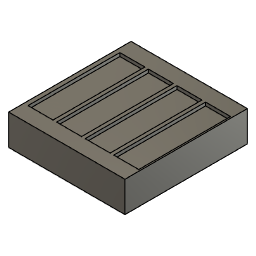
両端 v1 (Autodesk Fusion 360 design; units mm, degrees)
Autodesk Fusion 360 part; units mm, degrees
sketch "スケッチ1" plane through (0, 0, 0) normal (0, 1, 0) x (1, 0, 0)
  line L0 (0, 0) -> (-114, 0)
  line L1 (-114, 0) -> (-114, 120)
  line L2 (-114, 120) -> (0, 120)
  line L3 (0, 120) -> (0, 0)
  dimension "d1" = 114
  dimension "d2" = 120
  constraint horizontal L0
  constraint vertical L1
  constraint horizontal L2
  constraint vertical L3
  constraint coincident L0.start L3.end
  measures "d1" distance of L0.start L0.end
  measures "d2" distance of L0.start L2.end
extrude "押し出し1" add sketch "スケッチ1" along normal blind 40
sketch "スケッチ2" plane through (0, 40, 0) normal (0, 1, 0) x (-1, 0, 0)
  line L0 (0, -120) -> (114, -120)
  line L1 (114, -120) -> (114, 0)
  line L2 (114, 0) -> (0, 0)
  line L3 (0, 0) -> (0, -120)
  line L4 (0, -105) -> (1.5, -105)
  line L5 (1.5, -105) -> (1.5, -15)
  line L6 (1.5, -15) -> (0, -15)
  line L7 (0, -15) -> (0, -105)
  line L8 (1.5, -105) -> (26, -105)
  line L9 (26, -105) -> (26, -15)
  line L10 (26, -15) -> (1.5, -15)
  line L11 (1.5, -15) -> (1.5, -105)
  line L12 (26, -105) -> (29.5, -105)
  line L13 (29.5, -105) -> (29.5, -15)
  line L14 (29.5, -15) -> (26, -15)
  line L15 (26, -15) -> (26, -105)
  line L16 (29.5, -105) -> (54, -105)
  line L17 (54, -105) -> (54, -15)
  line L18 (54, -15) -> (29.5, -15)
  line L19 (29.5, -15) -> (29.5, -105)
  line L20 (54, -105) -> (57.5, -105)
  line L21 (57.5, -105) -> (57.5, -15)
  line L22 (57.5, -15) -> (54, -15)
  line L23 (54, -15) -> (54, -105)
  line L24 (57.5, -105) -> (82, -105)
  line L25 (82, -105) -> (82, -15)
  line L26 (82, -15) -> (57.5, -15)
  line L27 (57.5, -15) -> (57.5, -105)
  line L28 (82, -105) -> (85.5, -105)
  line L29 (85.5, -105) -> (85.5, -15)
  line L30 (85.5, -15) -> (82, -15)
  line L31 (82, -15) -> (82, -105)
  line L32 (85.5, -105) -> (110, -105)
  line L33 (110, -105) -> (110, -15)
  line L34 (110, -15) -> (85.5, -15)
  line L35 (85.5, -15) -> (85.5, -105)
  line L36 (110, -105) -> (114, -105)
  line L37 (114, -105) -> (114, -15)
  line L38 (114, -15) -> (110, -15)
  line L39 (110, -15) -> (110, -105)
  dimension "d5" = 1.5
  dimension "d6" = 90
  dimension "d7" = 24.5
  dimension "d8" = 90
  dimension "d9" = 3.5
  dimension "d10" = 90
  dimension "d11" = 24.5
  dimension "d12" = 90
  dimension "d13" = 3.5
  dimension "d14" = 90
  dimension "d15" = 24.5
  dimension "d16" = 90
  dimension "d17" = 3.5
  dimension "d18" = 90
  dimension "d19" = 24.5
  dimension "d20" = 90
  dimension "d21" = 4
  dimension "d22" = 90
  constraint horizontal L4
  constraint vertical L5
  constraint horizontal L6
  constraint vertical L7
  constraint coincident L3 L4.start
  constraint horizontal L8
  constraint vertical L9
  constraint horizontal L10
  constraint vertical L11
  constraint horizontal L12
  constraint vertical L13
  constraint horizontal L14
  constraint vertical L15
  constraint horizontal L16
  constraint vertical L17
  constraint horizontal L18
  constraint vertical L19
  constraint horizontal L20
  constraint vertical L21
  constraint horizontal L22
  constraint vertical L23
  constraint horizontal L24
  constraint vertical L25
  constraint horizontal L26
  constraint vertical L27
  constraint horizontal L28
  constraint vertical L29
  constraint horizontal L30
  constraint vertical L31
  constraint horizontal L32
  constraint vertical L33
  constraint horizontal L34
  constraint vertical L35
  constraint horizontal L36
  constraint vertical L37
  constraint horizontal L38
  constraint vertical L39
  measures "d5" distance of L4.start L4.end
  measures "d6" distance of L4.start L6.end
  measures "d7" distance of L4.end L8.end
  measures "d8" distance of L4.end L5.end
  measures "d9" distance of L8.end L12.end
  measures "d10" distance of L8.end L9.end
  measures "d11" distance of L12.end L16.end
  measures "d12" distance of L12.end L13.end
  measures "d13" distance of L16.end L20.end
  measures "d14" distance of L16.end L17.end
  measures "d15" distance of L20.end L24.end
  measures "d16" distance of L20.end L21.end
  measures "d17" distance of L24.end L28.end
  measures "d18" distance of L24.end L25.end
  measures "d19" distance of L28.end L32.end
  measures "d20" distance of L28.end L29.end
  measures "d21" distance of L32.end L36.end
  measures "d22" distance of L32.end L33.end
extrude "押し出し2" cut sketch "スケッチ2" against normal blind 3 contours L29 L32 L33 L34 L35 L39
sketch "スケッチ3" plane through (0, 40, 0) normal (0, 1, 0) x (-1, 0, 0)
  line L0 (110, -105) -> (85.5, -105)
  line L1 (85.5, -105) -> (85.5, -15)
  line L2 (85.5, -15) -> (110, -15)
  line L3 (110, -15) -> (110, -105)
  line L4 (0, -120) -> (114, -120)
  line L5 (114, -120) -> (114, 0)
  line L6 (114, 0) -> (0, 0)
  line L7 (0, 0) -> (0, -120)
  line L8 (0, -105) -> (1.5, -105)
  line L9 (1.5, -105) -> (1.5, -15)
  line L10 (1.5, -15) -> (0, -15)
  line L11 (0, -15) -> (0, -105)
  line L12 (1.5, -105) -> (26, -105)
  line L13 (26, -105) -> (26, -15)
  line L14 (26, -15) -> (1.5, -15)
  line L15 (1.5, -15) -> (1.5, -105)
  dimension "d25" = 1.5
  dimension "d26" = 90
  dimension "d27" = 24.5
  dimension "d28" = 90
  constraint horizontal L8
  constraint vertical L9
  constraint horizontal L10
  constraint vertical L11
  constraint coincident L7 L8.start
  constraint horizontal L12
  constraint vertical L13
  constraint horizontal L14
  constraint vertical L15
  measures "d25" distance of L8.start L8.end
  measures "d26" distance of L8.start L10.end
  measures "d27" distance of L8.end L12.end
  measures "d28" distance of L8.end L9.end
extrude "押し出し3" cut sketch "スケッチ3" against normal blind 3 contours L9 L12 L13 L14 L15
extrude "押し出し4" cut 1 faces at (-93.6667, 37, -45) along direction (0, -1, 0) blind 0.3
extrude "押し出し5" cut 1 faces at (-9.6667, 37, -45) along direction (0, -1, 0) blind 0.3
sketch "スケッチ4" plane through (0, 40, 0) normal (0, 1, 0) x (-1, 0, 0)
  line L0 (26, -105) -> (1.5, -105)
  line L1 (1.5, -105) -> (1.5, -15)
  line L2 (1.5, -15) -> (26, -15)
  line L3 (26, -15) -> (26, -105)
  line L4 (110, -105) -> (85.5, -105)
  line L5 (85.5, -105) -> (85.5, -15)
  line L6 (85.5, -15) -> (110, -15)
  line L7 (110, -15) -> (110, -105)
  line L8 (0, -120) -> (114, -120)
  line L9 (114, -120) -> (114, 0)
  line L10 (114, 0) -> (0, 0)
  line L11 (0, 0) -> (0, -120)
  line L12 (26, -105) -> (29.5, -105)
  line L13 (29.5, -105) -> (29.5, -15)
  line L14 (29.5, -15) -> (26, -15)
  line L15 (26, -15) -> (26, -105)
  line L16 (29.5, -105) -> (54, -105)
  line L17 (54, -105) -> (54, -15)
  line L18 (54, -15) -> (29.5, -15)
  line L19 (29.5, -15) -> (29.5, -105)
  dimension "d35" = 3.5
  dimension "d36" = 90
  dimension "d37" = 24.5
  dimension "d38" = 90
  constraint horizontal L12
  constraint vertical L13
  constraint horizontal L14
  constraint vertical L15
  constraint coincident L0.start L3.end
  constraint horizontal L16
  constraint vertical L17
  constraint horizontal L18
  constraint vertical L19
  measures "d35" distance of L0.start L12.end
  measures "d36" distance of L0.start L2.end
  measures "d37" distance of L12.end L16.end
  measures "d38" distance of L12.end L13.end
extrude "押し出し6" cut sketch "スケッチ4" against normal blind 3.3 contours L13 L16 L17 L18 L19
sketch "スケッチ5" plane through (0, 40, 0) normal (0, 1, 0) x (-1, 0, 0)
  line L0 (54, -105) -> (29.5, -105)
  line L1 (29.5, -105) -> (29.5, -15)
  line L2 (29.5, -15) -> (54, -15)
  line L3 (54, -15) -> (54, -105)
  line L4 (26, -105) -> (1.5, -105)
  line L5 (1.5, -105) -> (1.5, -15)
  line L6 (1.5, -15) -> (26, -15)
  line L7 (26, -15) -> (26, -105)
  line L8 (110, -105) -> (85.5, -105)
  line L9 (85.5, -105) -> (85.5, -15)
  line L10 (85.5, -15) -> (110, -15)
  line L11 (110, -15) -> (110, -105)
  line L12 (0, -120) -> (114, -120)
  line L13 (114, -120) -> (114, 0)
  line L14 (114, 0) -> (0, 0)
  line L15 (0, 0) -> (0, -120)
  line L16 (54, -105) -> (57.5, -105)
  line L17 (57.5, -105) -> (57.5, -15)
  line L18 (57.5, -15) -> (54, -15)
  line L19 (54, -15) -> (54, -105)
  line L20 (57.5, -105) -> (82, -105)
  line L21 (82, -105) -> (82, -15)
  line L22 (82, -15) -> (57.5, -15)
  line L23 (57.5, -15) -> (57.5, -105)
  dimension "d41" = 3.5
  dimension "d42" = 90
  dimension "d43" = 24.5
  dimension "d44" = 90
  constraint horizontal L16
  constraint vertical L17
  constraint horizontal L18
  constraint vertical L19
  constraint coincident L0.start L3.end
  constraint horizontal L20
  constraint vertical L21
  constraint horizontal L22
  constraint vertical L23
  measures "d41" distance of L0.start L16.end
  measures "d42" distance of L0.start L2.end
  measures "d43" distance of L16.end L20.end
  measures "d44" distance of L16.end L17.end
extrude "押し出し7" cut sketch "スケッチ5" against normal blind 3.3 contours L17 L20 L21 L22 L23
extrude "押し出し8" cut 4 faces at (-93.6667, 36.7, -45) (-65.6667, 36.7, -45) (-37.6667, 36.7, -45) (-9.6667, 36.7, -45) along direction (0, -1, 0) blind 10
extrude "押し出し9" cut 1 faces at (-57.1667, 40, -5) along direction (0, -1, 0) blind 10
